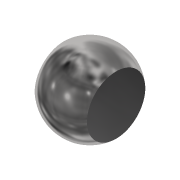
# Autodesk Inventor part: Rocker Box Ball
Saved by Autodesk Inventor 2014 (Build 180170000, 170)
## iProperties
Created: 2013-05-18
Part Number: Rocker Box Ball
Material: Stainless Steel
Document SubType Name: Modeling
Designer: richard
Density: 8.08 g/cm^3
Appearance: Steel - Polished
Author: richard
Autodesk Inventor part; units mm, degrees
ref_plane "YZ Plane" through (0, 0, 0) normal (1, 0, 0) x (0, 1, 0)
ref_plane "XZ Plane" through (0, 0, 0) normal (0, 1, 0) x (-1, 0, 0)
ref_plane "XY Plane" through (0, 0, 0) normal (0, 0, 1) x (1, 0, 0)
sketch "Sketch1" plane through (0, 0, 0) normal (0, 0, 1) x (1, 0, 0)
  line L0 (-10, 0) -> (10, 0)
  arc A0 (10, 11.1803) -> (-10, 11.1803) centre (0, 0) ccw
  line L1 (-10, 0) -> (-10, 11.1803)
  line L2 (10, 0) -> (10, 11.1803)
  line L3 (0, 0) -> (0, 15) construction
  dimension "d1" = 15
  dimension "d2" = 20
  constraints: 8 end point, 3 point on circle, 2 midpoint, 2 parallel, 1 centre point, 1 coincident, 1 horizontal, 1 perpendicular, 1 other
  measures "d1" radius of A0
  measures "d2" distance of L0.start L0.end
revolve "Revolution1" add sketch "Sketch1" angle 360 about axis through (-10, 0, 0) along (1, 0, 0)
sketch "Sketch2" plane through (10, 0, 0) normal (1, 0, 0) x (0, 0, -1)
  circle A0 centre (0, 0) radius 11.1803 projected
  line L0 (8, -4) -> (-8, -4)
  line L1 (-8, -4) -> (-8, 4)
  line L2 (-8, 4) -> (8, 4)
  line L3 (8, 4) -> (8, -4)
  line L4 (8, -4) -> (-8, 4) construction
  line L5 (-8, -4) -> (8, 4) construction
  dimension "d4" = 8
  dimension "d5" = 16
  constraints: 12 end point, 2 midpoint, 2 parallel, 1 horizontal, 1 perpendicular
  measures "d4" distance of L0.end L1.end
  measures "d5" distance of L1.end L2.end
extrude "Extrusion1" [suppressed]
body "Solid1"
